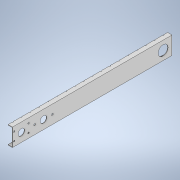
# Autodesk Inventor part: VerseFrame 18in C Channel
Saved by Autodesk Inventor 2021 (Build 250183000, 183)
## iProperties
Created: 2020-01-13
Part Number: VerseFrame 18in C Channel
Material: Generic
Document SubType Name: Modeling
Designer: aidan
Density: 1 g/cm^3
Appearance: Default
Author: aidan
Autodesk Inventor part; units mm, degrees
ref_plane "YZ Plane" through (0, 0, 0) normal (1, 0, 0) x (0, 1, 0)
ref_plane "XZ Plane" through (0, 0, 0) normal (0, 1, 0) x (-1, 0, 0)
ref_plane "XY Plane" through (0, 0, 0) normal (0, 0, 1) x (1, 0, 0)
sketch "Sketch1" plane through (0, 0, 0) normal (0, 0, 1) x (1, 0, 0)
  line L0 (-12.1708, 16.0073) -> (13.2292, 16.0073)
  line L1 (13.2292, 16.0073) -> (13.2292, -34.7927)
  line L2 (13.2292, -34.7927) -> (-12.1708, -34.7927)
  line L3 (-12.1708, -34.7927) -> (-12.1708, 16.0073)
  line L4 (11.9592, 14.7373) -> (-10.9008, 14.7373)
  line L5 (-10.9008, 14.7373) -> (-10.9008, -33.5227)
  line L6 (-10.9008, -33.5227) -> (11.9592, -33.5227)
  line L7 (11.9592, -33.5227) -> (11.9592, 14.7373)
  point P0 (0, 0)
  dimension "d0" = 25.4
  dimension "d1" = 50.8
  dimension "d2" = 1.27
  constraints: 16 end point, 4 parallel, 2 perpendicular, 1 horizontal, 3 other
  measures "d0" distance of L0.start L0.end
  measures "d1" distance of L0.end L1.end
  measures "d2" distance between parallel lines of L0 L4
extrude "Extrusion1" add sketch "Sketch1" along normal blind 457.2
sketch "Sketch2" plane through (-12.1708, 16.0073, 0) normal (0, 1, 0) x (1, 0, 0)
  circle A0 centre (12.7, -12.7) radius 1.7272
  line L0 (25.4, 0) -> (0, 0) projected
  line L1 (0, 0) -> (0, -457.2) projected
  point P0 (12.1708, 0)
  dimension "d5" = 3.4544
  dimension "d6" = 12.7
  dimension "d7" = 12.7
  constraints: 1 centre point
  measures "d5" diameter of A0
  measures "d6" distance from line of L0 A0.centre
  measures "d7" distance from line of L1 A0.centre
extrude "Extrusion2" cut sketch "Sketch2" against normal through all
pattern_linear "Rectangular Pattern1" count 46 spacing 25.4 along (0, 0, 1) of "Extrusion2"
sketch "Sketch3" plane through (0, 0, 457.2) normal (0, 0, 1) x (1, 0, 0)
  line L0 (-12.1708, 16.0073) -> (-12.1708, -34.7927) projected
  line L1 (-12.1708, -34.7927) -> (13.2292, -34.7927) projected
  line L2 (-12.1708, 16.0073) -> (0.5292, 16.0073)
  line L3 (0.5292, 16.0073) -> (0.5292, -34.7927)
  line L4 (0.5292, -34.7927) -> (-12.1708, -34.7927)
  line L5 (-12.1708, -34.7927) -> (-12.1708, 16.0073)
  line L6 (11.9592, -33.5227) -> (-10.9008, -33.5227) projected
  line L7 (-10.9008, -33.5227) -> (-10.9008, 14.7373) projected
  line L8 (0.5292, -33.5227) -> (-10.9008, -33.5227)
  line L9 (-10.9008, -33.5227) -> (-10.9008, 14.7373)
  line L10 (-10.9008, 14.7373) -> (0.5292, 14.7373)
  line L11 (0.5292, 14.7373) -> (0.5292, -33.5227)
  point P0 (0, 0)
  point P1 (0.5292, -33.5227)
  dimension "d15" = 12.7
  constraints: 16 end point, 4 parallel, 2 horizontal, 2 midpoint, 2 perpendicular
  measures "d15" distance of L0.start L2.end
extrude "Extrusion3" cut sketch "Sketch3" against normal blind 457.2 contours L2 L3 L10 L7 L6 L1 L0
sketch "Sketch4" plane through (13.2292, -34.7927, 0) normal (1, 0, 0) x (0, 0, -1)
  line L0 (-457.2, 0) -> (-457.2, 50.8) projected
  line L1 (-457.2, 25.4) -> (0, 25.4) construction
  line L2 (0, 0) -> (0, 50.8) projected
  circle A0 centre (-431.8, 25.4) radius 9.525
  circle A1 centre (-368.3, 25.4) radius 9.525
  circle A2 centre (-393.7, 25.4) radius 2.5781
  circle A3 centre (-342.9, 25.4) radius 2.5781
  circle A4 centre (-368.3, 25.4) radius 25.4 construction
  circle A5 centre (-25.4, 25.4) radius 14.2875
  line L3 (-452.4222, 13.4938) -> (-411.1778, 13.4938) construction
  line L4 (-411.1778, 13.4938) -> (-411.1778, 37.3063) construction
  line L5 (-411.1778, 37.3063) -> (-452.4222, 37.3063) construction
  line L6 (-452.4222, 37.3063) -> (-452.4222, 13.4938) construction
  line L7 (-452.4222, 13.4938) -> (-411.1778, 37.3063) construction
  line L8 (-411.1778, 13.4938) -> (-452.4222, 37.3063) construction
  point P0 (0, 34.7927)
  dimension "d18" = 28.575
  dimension "d19" = 50.8
  dimension "d20" = 5.1562
  dimension "d21" = 19.05
  dimension "d22" = 25.4
  dimension "d23" = 25.4
  dimension "d24" = 19.05
  dimension "d25" = 63.5
  dimension "d26" = 47.625
  dimension "d27" = 60
  constraints: 14 end point, 6 centre point, 5 point on line, 4 midpoint, 2 horizontal, 2 parallel, 2 point on circle, 1 coincident, 1 equal radius, 1 perpendicular
  measures "d18" diameter of A5
  measures "d19" diameter of A4
  measures "d20" diameter of A3
  measures "d21" diameter of A1
  measures "d22" distance from line of L0 A0.centre
  measures "d23" distance from line of L2 A5.centre
  measures "d24" diameter of A0
  measures "d25" distance of A1.centre A0.centre
  measures "d26" distance of L3.end L5.end
  measures "d27" angle of L7 L8
extrude "Extrusion4" cut sketch "Sketch4" against normal through all
sketch "Sketch5" plane through (13.2292, -34.7927, 0) normal (1, 0, 0) x (0, 0, -1)
  circle A0 centre (-431.8, 25.4) radius 9.525 projected
  circle A1 centre (-431.8, 25.4) radius 23.8125 construction
  line L0 (-452.4222, 37.3062) -> (-411.1778, 13.4937) construction
  line L1 (-452.4222, 13.4938) -> (-411.1778, 37.3063) construction
  line L2 (0, 0) -> (-457.2, 0) projected
  circle A2 centre (-452.4222, 37.3062) radius 2.1463
  circle A3 centre (-411.1778, 37.3063) radius 2.1463
  circle A4 centre (-411.1778, 13.4937) radius 2.1463
  circle A5 centre (-452.4222, 13.4938) radius 2.1463
  point P0 (0, 34.7927)
  point P1 (-431.8, 25.4)
  dimension "d30" = 47.625
  dimension "d31" = 60
  dimension "d32" = 30
  dimension "d33" = 4.2926
  constraints: 5 centre point, 5 coincident, 4 end point, 4 point on circle, 3 equal radius, 3 midpoint
  measures "d30" diameter of A1
  measures "d31" angle of L1 L0
  measures "d32" angle of L2 L1
  measures "d33" diameter of A2
extrude "Extrusion5" cut sketch "Sketch5" against normal through all contours A2 | A3 | A4 | A5
equation "\"d3\" = d13"
equation "\"d16\" = d13"
equation "\"d14\" = d13"
equation "\"d10\" = d14"
equation "\"d13\" = 457.2"
body "Solid1"
